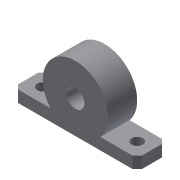
# Autodesk Inventor part: 00_spindel_bearings
Saved by Autodesk Inventor 2019.4 (Build 234330000, 330)
## iProperties
Created: 2020-10-27
Part Number: 00_spindel_bearings
Material: Generic
Document SubType Name: Modeling
Designer: diederichbenedict
Density: 1 g/cm^3
Appearance: Default
Author: diederichbenedict
Autodesk Inventor part; units mm, degrees
ref_plane "YZ Plane" through (0, 0, 0) normal (1, 0, 0) x (0, 1, 0)
ref_plane "XZ Plane" through (0, 0, 0) normal (0, 1, 0) x (-1, 0, 0)
ref_plane "XY Plane" through (0, 0, 0) normal (0, 0, 1) x (1, 0, 0)
sketch "Sketch1" plane through (0, 0, 0) normal (0, 0, 1) x (1, 0, 0)
  circle A0 centre (0, 0) radius 4
  circle A1 centre (0, 0) radius 14.5
  line L0 (-27.5, -14.5) -> (27.5, -14.5)
  line L1 (27.5, -14.5) -> (27.5, -9.31)
  line L2 (27.5, -9.31) -> (-27.5, -9.31)
  line L3 (-27.5, -9.31) -> (-27.5, -14.5)
  dimension "d0" = 8
  dimension "d1" = 29
  dimension "d2" = 27.5
  dimension "d3" = 27.5
  dimension "d4" = 5.19
  constraints: 8 end point, 2 centre point, 2 coincident, 2 parallel, 1 horizontal, 1 perpendicular
  measures "d0" diameter of A0
  measures "d1" diameter of A1
  measures "d2" distance from line of L3 point (0, 0)
  measures "d3" distance from line of L1 point (0, 0)
  measures "d4" distance between parallel lines of L0 L2
extrude "Extrusion1" add sketch "Sketch1" along normal blind 13
sketch "Sketch2" plane through (11.1164, -9.31, 0) normal (0, 1, 0) x (1, 0, 0)
  line L0 (-22.2328, -13) -> (-22.2328, 0) projected
  line L1 (-22.2328, 0) -> (-38.6164, 0) projected
  line L2 (-38.6164, 0) -> (-38.6164, -13) projected
  line L3 (-22.2328, -13) -> (-38.6164, -13) projected
  line L4 (0, 0) -> (0, -13) projected
  line L5 (16.3836, -13) -> (0, -13) projected
  line L6 (16.3836, 0) -> (16.3836, -13) projected
  line L7 (16.3836, 0) -> (0, 0) projected
  circle A0 centre (-32.1164, -6.5) radius 2.5
  circle A1 centre (9.8836, -6.5) radius 2.5
  line L8 (0, 0) -> (0, -13) projected
  line L9 (-22.2328, 0) -> (0, 0) projected
  line L10 (-22.2328, -13) -> (-22.2328, 0) projected
  line L11 (0, -13) -> (-22.2328, -13) projected
  point P0 (-11.1164, 0)
  dimension "d7" = 5
  dimension "d8" = 5
  dimension "d9" = 21
  dimension "d10" = 21
  constraints: 2 centre point
  measures "d7" diameter of A0
  measures "d8" diameter of A1
  measures "d9" horizontal distance of point (-11.116, 0) A0.centre
  measures "d10" horizontal distance of A1.centre point (-11.116, 0)
extrude "Extrusion2" cut sketch "Sketch2" against normal through all contours A0 | A1
chamfer "Chamfer1" distance 2 angle 45 4 edges at (-27.5, -11.905, 0) (27.5, -11.905, 0) (27.5, -11.905, 13) (-27.5, -11.905, 13)
body "Solid1"
